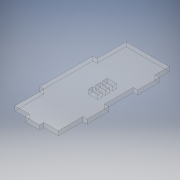
# Autodesk Inventor part: top_right_v2
Saved by Autodesk Inventor 2017.2 (Build 212233000, 233)
## iProperties
Created: 2017-06-09
Part Number: top_right_v2
Material: Generic
Document SubType Name: Modeling
Designer: SandeepSH
Density: 1 g/cm^3
Appearance: Polycarbonate - Clear
Author: SandeepSH
Autodesk Inventor part; units mm, degrees
ref_plane "YZ Plane" through (0, 0, 0) normal (1, 0, 0) x (0, 1, 0)
ref_plane "XZ Plane" through (0, 0, 0) normal (0, 1, 0) x (-1, 0, 0)
ref_plane "XY Plane" through (0, 0, 0) normal (0, 0, 1) x (1, 0, 0)
sketch "Sketch1" plane through (0, 0, 0) normal (0, 1, 0) x (-1, 0, 0)
  line L0 (0, 0) -> (-36, 0)
  line L1 (-36, 0) -> (-36, -80)
  line L2 (-36, -80) -> (0, -80)
  line L3 (0, -80) -> (0, 0)
  dimension "d0" = 36
  dimension "d1" = 80
  constraints: 8 end point, 2 parallel, 1 horizontal, 1 perpendicular
  measures "d0" distance of L2.end L1.end
  measures "d1" distance of L1.end L0.end
extrude "Extrusion1" add sketch "Sketch1" along normal blind 3
sketch "Sketch2" plane through (0, 3, 0) normal (0, 1, 0) x (1, 0, 0)
  line L0 (0, 0) -> (36, 0) projected
  line L1 (36, 0) -> (23, 0)
  line L2 (23, 0) -> (23, 3)
  line L3 (23, 3) -> (36, 3)
  line L4 (36, 3) -> (36, 0)
  line L5 (0, 0) -> (13, 0)
  line L6 (13, 0) -> (13, 3)
  line L7 (13, 3) -> (0, 3)
  line L8 (0, 3) -> (0, 0)
  line L9 (0, 3) -> (3, 3)
  line L10 (3, 3) -> (3, 23)
  line L11 (3, 23) -> (0, 23)
  line L12 (0, 23) -> (0, 3)
  line L13 (36, 80) -> (0, 80) projected
  line L14 (0, 80) -> (3, 80)
  line L15 (3, 80) -> (3, 60)
  line L16 (3, 60) -> (0, 60)
  line L17 (0, 60) -> (0, 80)
  line L18 (36, 3) -> (33, 3)
  line L19 (33, 3) -> (33, 20)
  line L20 (33, 20) -> (36, 20)
  line L21 (36, 20) -> (36, 3)
  line L22 (36, 0) -> (36, 80) projected
  line L23 (36, 35) -> (33, 35)
  line L24 (33, 35) -> (33, 55)
  line L25 (33, 55) -> (36, 55)
  line L26 (36, 55) -> (36, 35)
  line L27 (36, 80) -> (33, 80)
  line L28 (33, 80) -> (33, 70)
  line L29 (33, 70) -> (36, 70)
  line L30 (36, 70) -> (36, 80)
  dimension "d4" = 13
  dimension "d5" = 3
  dimension "d6" = 3
  dimension "d7" = 10
  dimension "d8" = 3
  dimension "d9" = 20
  dimension "d10" = 3
  dimension "d11" = 20
  dimension "d12" = 3
  dimension "d13" = 17
  dimension "d14" = 3
  dimension "d15" = 20
  dimension "d16" = 15
  dimension "d17" = 3
  dimension "d18" = 15
  constraints: 56 end point, 14 parallel, 7 horizontal, 7 perpendicular, 1 point on line
  measures "d4" distance of L2.end L3.end
  measures "d5" distance of L1.end L2.end
  measures "d6" distance of L6.end L5.end
  measures "d7" distance between parallel lines of L2 L6
  measures "d8" distance of L11.end L10.end
  measures "d9" distance of L10.end L9.end
  measures "d10" distance of L15.end L16.end
  measures "d11" distance of L14.end L15.end
  measures "d12" distance of L19.end L20.end
  measures "d13" distance of L18.end L19.end
  measures "d14" distance of L24.end L25.end
  measures "d15" distance of L23.end L24.end
  measures "d16" distance between parallel lines of L23 L20
  measures "d17" distance of L29.end L28.end
  measures "d18" distance between parallel lines of L25 L29
extrude "Extrusion2" cut sketch "Sketch2" against normal through all
sketch "Sketch3" plane through (0, 3, 0) normal (0, 1, 0) x (1, 0, 0)
  line L0 (0, 51.5) -> (18.5, 51.5)
  line L1 (18.5, 51.5) -> (18.5, 38.5)
  line L2 (18.5, 38.5) -> (0, 38.5)
  line L3 (0, 38.5) -> (0, 51.5)
  line L4 (13, 0) -> (23, 0) projected
  line L5 (18.5, 38.5) -> (25, 38.5)
  line L6 (25, 38.5) -> (25, 41.5)
  line L7 (25, 41.5) -> (18.5, 41.5)
  line L8 (18.5, 41.5) -> (18.5, 38.5)
  line L9 (18.5, 51.5) -> (25, 51.5)
  line L10 (25, 51.5) -> (25, 48.5)
  line L11 (25, 48.5) -> (18.5, 48.5)
  line L12 (18.5, 48.5) -> (18.5, 51.5)
  line L13 (18.5, 46.5) -> (25, 46.5)
  line L14 (25, 46.5) -> (25, 43.5)
  line L15 (25, 43.5) -> (18.5, 43.5)
  line L16 (18.5, 43.5) -> (18.5, 46.5)
  point P0 (0, 0)
  dimension "d21" = 18.5
  dimension "d22" = 13
  dimension "d23" = 38.5
  dimension "d24" = 6.5
  dimension "d25" = 3
  dimension "d26" = 6.5
  dimension "d27" = 3
  dimension "d28" = 6.5
  dimension "d29" = 3
  dimension "d30" = 2
  constraints: 32 end point, 8 parallel, 4 horizontal, 4 perpendicular, 1 point on line
  measures "d21" distance of L1.end L2.end
  measures "d22" distance of L0.end L1.end
  measures "d23" distance between parallel lines of L4 L2
  measures "d24" distance of L7.end L6.end
  measures "d25" distance of L6.end L5.end
  measures "d26" distance of L10.end L11.end
  measures "d27" distance of L9.end L10.end
  measures "d28" distance between parallel lines of L14 L16
  measures "d29" distance between parallel lines of L13 L15
  measures "d30" distance between parallel lines of L7 L15
extrude "Extrusion3" cut sketch "Sketch3" against normal through all contours L9 L10 L11 L1 | L1 L7 L6 L5 | L13 L14 L15 L1
equation "\"d28\" = d24"
equation "\"d29\" = d27"
body "Solid1"
